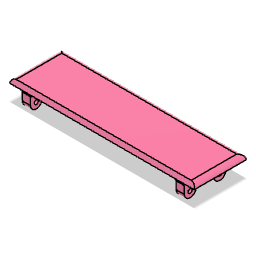
Panneau Supérieur (Autodesk Fusion 360 design; units mm, degrees)
Autodesk Fusion 360 part; units mm, degrees
sketch "Dessus" plane through (71.9136, 0, 0) normal (1, 0, 0) x (0, 0, -1)
  line L0 (-29.5234, 102.1046) -> (-29.5234, 98.9121)
  line L1 (-29.5234, 98.9121) -> (-27.1828, 99.764)
  line L2 (-27.1828, 99.764) -> (2.7408, 181.9785)
  line L3 (2.7408, 181.9785) -> (-0.4517, 181.9785)
  line L4 (-0.4517, 181.9785) -> (-29.5234, 102.1046)
  line L5 (2.7408, 181.9785) -> (33.8089, 181.9785)
  line L6 (1.6489, 178.9785) -> (33.8089, 178.9785)
  line L7 (30.8089, 189.0529) -> (30.8089, 172.1154) construction
  line L8 (30.8089, 0) -> (30.8089, 3) construction
  line L9 (33.8089, 181.9785) -> (33.8089, 178.9785)
  line L10 (33.8089, 187.4367) -> (33.8089, 173.0665) construction
  dimension "d170" = 3
  dimension "d276" = 3
  constraint coincident L2.end L3.start
  constraint parallel L3 L5
  constraint coincident L2 L6.start
  constraint parallel L5 L6
  constraint vertical L7
  constraint collinear L7 L8
  constraint vertical L10
  constraint collinear L9 L10
  measures "d170" distance of L5 L6
  measures "d276" distance of L7 L10
extrude "Extrude1" add sketch "Dessus" against normal blind 114 contours L2 L5 L6 L9
ref_plane "WorkPlane1" through (64.9136, 180.4785, -17.7289) normal (1, 0, 0) x (0, 0, -1)
sketch "Fixations" plane through (64.9136, 180.4785, -16.2289) normal (1, 0, 0) x (0, 0, -1)
  circle A0 centre (-10.1337, -7.85) radius 1.25
  line L0 (-12.7166, -11.5) -> (1.5244, -11.5) construction
  line L1 (-5.1603, -4.8175) -> (-5.1603, -4.8577) construction
  line L2 (-5.1603, -4.8577) -> (-8.0065, -12.6776) construction
  line L3 (-43.4117, -80.7145) -> (-13.4881, 1.5) construction
  line L4 (-14.58, -1.5) -> (17.58, -1.5) construction
  circle A1 centre (-10.1337, -7.85) radius 3.65
  line L5 (-6.4837, -1.5) -> (-6.4837, -10.4978)
  line L6 (-13.7837, -1.5) -> (-6.4837, -1.5)
  line L7 (-14.58, -1.5) -> (-6.4837, -1.5)
  line L8 (-13.7837, -1.5) -> (-13.7837, -9.2816)
  line L9 (4.58, -1.5) -> (4.58, -10.0199)
  line L10 (17.58, 1.5) -> (17.58, -1.5) construction
  line L11 (6.1114, -11.5) -> (14.8051, -11.5) construction
  circle A2 centre (8.23, -7.85) radius 1.25
  circle A3 centre (8.23, -7.85) radius 3.65
  line L12 (11.88, -1.5) -> (11.88, -9.9125)
  line L13 (11.88, -1.5) -> (4.58, -1.5)
  dimension "d174" = 2.5
  dimension "d175" = 10
  dimension "d176" = 10
  dimension "d177" = 2.4
  dimension "d183" = 13
  dimension "d184" = 10
  dimension "d185" = 2.5
  dimension "d186" = 2.4
  constraint horizontal L0
  constraint perpendicular L0 L1
  constraint parallel L2 L3
  constraint tangent L2 A1
  constraint tangent L0 A1
  constraint coincident L4 L5.start
  constraint perpendicular L4 L5
  constraint coincident L4 L6.start
  constraint tangent A1 L5
  constraint coincident L4.start L7.start
  constraint coincident L7 L6.start
  constraint perpendicular L7 L8
  constraint tangent A1 L8
  constraint vertical L9
  constraint horizontal L11
  constraint tangent L9 A3
  constraint tangent L11 A3
  constraint coincident L4 L12.start
  constraint perpendicular L4 L12
  constraint coincident L4 L9.start
  constraint tangent A3 L12
  measures "d174" diameter of A0
  measures "d175" distance of L0 L4
  measures "d176" distance of L2 L3
  measures "d183" distance of L9 L10
  measures "d184" distance of L4 L11
  measures "d185" diameter of A2
extrude "Extrude2" add sketch "Fixations" against normal blind 5
fillet "Fillet1" radius 2 2 edges at (62.4136, 178.9785, -9.7452) (59.9136, 178.9785, -6.0952)
fillet "Fillet1" radius 2 1 edges at (62.4136, 178.9785, -2.4452)
fillet "Fillet1" radius 2 3 edges at (62.4136, 178.9785, -20.8089) (62.4136, 178.9785, -28.1089) (59.9136, 178.9785, -24.4589)
ref_plane "WorkPlane2" through (14.9136, 180.4785, -17.7289) normal (1, 0, 0) x (0, 0, -1)
mirror "Mirror1" about plane through (14.9136, 180.4785, -17.7289) normal (1, 0, 0) of "Extrude2", "Fillet1"
fillet "Fillet2" radius 3 3 edges at (-42.0864, 181.9785, -18.2748) (14.9136, 181.9785, -33.8089) (71.9136, 181.9785, -18.2748)
sketch "Sketch3" plane through (-39.0864, 0, 0) normal (1, 0, 0) x (0, 0, -1)
  circle A0 centre (-12.2411, 48.3) radius 3
  circle A1 centre (-121.8411, 48.35) radius 1.5
  circle A2 centre (24.4589, 172.6285) radius 1.5
  circle A3 centre (6.0952, 172.6285) radius 1.5
  circle A4 centre (-50.9889, 84.3418) radius 1.5
  circle A5 centre (24.4589, 89.4893) radius 1.5
  circle A6 centre (-103.3298, 65.2912) radius 1.5
  circle A7 centre (-121.8411, 9.35) radius 1.5
  circle A8 centre (-19.9674, 101.0221) radius 1.5
  circle A9 centre (24.4589, 9.35) radius 1.5
  line L0 (30.8089, 0) -> (30.8089, 178.9785)
  line L1 (30.8089, 178.9785) -> (1.6489, 178.9785)
  line L2 (1.6489, 178.9785) -> (-27.1828, 99.764)
  line L3 (-27.1828, 99.764) -> (-128.1911, 63)
  line L4 (-128.1911, 63) -> (-128.1911, 0)
  line L5 (-128.1911, 0) -> (30.8089, 0)
  circle A10 centre (-72.2411, 48.3) radius 3
  line L6 (-86.4911, 47.6165) -> (-86.4911, 22.0965) construction
  dimension "d300" = 117.3
  constraint vertical L6
  measures "d300" distance of L0 L6
equation "d170 = EpaisseurParoi"
equation "d171 = -Largeur - 2 * EpaisseurParoi"
equation "d173 = -EpaisseurParoi - Tolerance - 3 mm - Tolerance"
equation "d174 = PerçageO3"
equation "d177 = EpaisseurParoiPerçage"
equation "d183 = 10 mm + EpaisseurParoi"
equation "d185 = PerçageO3"
equation "d186 = EpaisseurParoiPerçage"
equation "d276 = EpaisseurParoi"
equation "d280 = EpaisseurParoi"
equation "d300 = 120.3 mm - EpaisseurParoi"
equation "Largeur = 108 mm"
equation "EpaisseurParoi = 3 mm"
equation "Tolerance = 0.5 mm"
equation "PerçageO3 = 2.5 mm"
equation "EpaisseurParoiPerçage = 2.4 mm"
